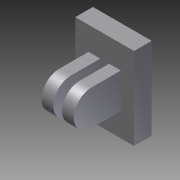
# Autodesk Inventor part: piston mount bracket
Saved by Autodesk Inventor 2012 (Build 160160000, 160)
## iProperties
Created: 2011-12-02
Part Number: piston mount bracket
Material: Default
Document SubType Name: Modeling
Designer: Antonella
Density: 1 g/cm^3
Author: Antonella
Autodesk Inventor part; units mm, degrees
ref_plane "YZ Plane" through (0, 0, 0) normal (1, 0, 0) x (0, 1, 0)
ref_plane "XZ Plane" through (0, 0, 0) normal (0, 1, 0) x (-1, 0, 0)
ref_plane "XY Plane" through (0, 0, 0) normal (0, 0, 1) x (1, 0, 0)
sketch "Sketch1" plane through (0, 0, 0) normal (0, 0, 1) x (1, 0, 0)
  line L0 (-11.1125, 0) -> (11.1125, 0) projected
  line L1 (0, -15.5575) -> (0, 15.5575) projected
  line L2 (-7.9375, 11.1125) -> (7.9375, 11.1125)
  line L3 (7.9375, 11.1125) -> (7.9375, -11.1125)
  line L4 (7.9375, -11.1125) -> (-7.9375, -11.1125)
  line L5 (-7.9375, -11.1125) -> (-7.9375, 11.1125)
  point P0 (0, 0)
  point P1 (-7.9375, 0)
  point P2 (0, 11.1125)
  dimension "d0" = 15.875
  dimension "d1" = 22.225
  constraints: 8 end point, 2 midpoint, 2 parallel, 1 horizontal, 1 horizontal alignment, 1 perpendicular, 1 vertical alignment
  measures "d0" distance of L2.start L2.end
  measures "d1" distance of L4.end L2.start
extrude "Extrusion1" add sketch "Sketch1" along normal blind 4.7625
sketch "Sketch2" plane through (0, 0, 4.7625) normal (0, 0, 1) x (1, 0, 0)
  line L0 (4.3656, 4.7625) -> (4.3656, -4.7625)
  line L1 (-4.3656, -4.7625) -> (-4.3656, 4.7625)
  line L2 (-1.1906, 4.7625) -> (-1.1906, -4.7625)
  line L3 (1.1906, 4.7625) -> (1.1906, -4.7625)
  line L4 (-4.3656, 4.7625) -> (-1.1906, 4.7625)
  line L5 (1.1906, 4.7625) -> (4.3656, 4.7625)
  line L6 (4.3656, -4.7625) -> (1.1906, -4.7625)
  line L7 (-1.1906, -4.7625) -> (-4.3656, -4.7625)
  line L8 (1.1906, 4.7625) -> (-1.1906, 4.7625) construction
  line L9 (-1.1906, -4.7625) -> (1.1906, -4.7625) construction
  point P0 (0, 0)
  point P1 (-4.3656, 0)
  point P2 (0, 6.35)
  point P3 (0, 4.7625)
  dimension "d5" = 9.525
  dimension "d10" = 2.3813
  dimension "d11" = 3.175
  constraints: 20 end point, 6 parallel, 6 perpendicular, 2 collinear, 2 horizontal, 2 midpoint, 2 vertical alignment, 1 horizontal alignment
  measures "d5" distance of L1.start L1.end
  measures "d10" distance between parallel lines of L2 L3
  measures "d11" distance of L3.start L0.start
extrude "Extrusion4" add sketch "Sketch2" along normal blind 12.7
sketch "Sketch4" plane through (4.3656, -4.7625, 4.7625) normal (1, 0, 0) x (0, 0, -1)
  line L0 (-12.7, 9.525) -> (-12.7, 0) projected
  line L1 (0, 0) -> (-12.7, 0) projected
  line L2 (0, 9.525) -> (0, 0) projected
  line L3 (0, 9.525) -> (-12.7, 9.525) projected
  arc A0 (-7.9375, 9.525) -> (-7.9375, 0) centre (-7.9375, 4.7625) ccw
  point P0 (4.7625, 4.7625)
  constraints: 3 tangent, 2 point on circle, 2 point on line, 1 centre point
extrude "Extrusion5" cut sketch "Sketch4" against normal through all contours L3 A0 L0 | A0 L1 L0
body "Solid1"
